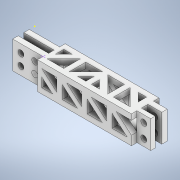
# Autodesk Inventor part: Final design
Saved by Autodesk Inventor 2021 (Build 250183000, 183)
## iProperties
Created: 2021-03-23
Part Number: Final design
Material: ABS Plastic
Document SubType Name: Modeling
Designer: kcf23
Mass: 34.1575 g
Surface Area: 224.112 cm^2
Volume: 32.224 cm^3
Density: 1.06 g/cm^3
Appearance: Smooth - White
Author: kcf23
Autodesk Inventor part; units mm, degrees
ref_plane "YZ Plane" through (0, 0, 0) normal (1, 0, 0) x (0, 1, 0)
ref_plane "XZ Plane" through (0, 0, 0) normal (0, 1, 0) x (-1, 0, 0)
ref_plane "XY Plane" through (0, 0, 0) normal (0, 0, 1) x (1, 0, 0)
sketch "Sketch1" plane through (0, 0, 0) normal (0, 0, 1) x (1, 0, 0)
  line L0 (0, 0) -> (127, 0)
  line L1 (127, 0) -> (127, 25.4)
  line L2 (127, 25.4) -> (0, 25.4)
  line L3 (0, 25.4) -> (0, 0)
  line L4 (0, 0) -> (12.7, 0)
  line L5 (12.7, 25.4) -> (0, 25.4)
  line L6 (0, 25.4) -> (0, 0)
  line L7 (7.62, 25.4) -> (0, 25.4)
  line L8 (0, 25.4) -> (0, -8.7611)
  line L9 (125.2545, 0) -> (125.2545, 25.4)
  circle A0 centre (121.4445, 4.9881) radius 2.2479
  circle A1 centre (121.4445, 12.6081) radius 2.2479
  circle A2 centre (121.4445, 20.2281) radius 2.2479
  line L10 (125.2545, 0) -> (117.6345, 0)
  line L11 (117.6345, 0) -> (117.6345, 25.4)
  line L12 (125.2545, 25.4) -> (117.6345, 25.4)
  line L13 (21.1145, 0) -> (21.1145, 25.4)
  circle A3 centre (5.08, 6.985) radius 2.2479
  line L14 (5.08, 6.985) -> (17.78, 6.985)
  circle A4 centre (17.78, 6.985) radius 2.2479
  circle A5 centre (5.08, 19.05) radius 2.2479
  line L15 (5.08, 19.05) -> (17.78, 19.05)
  circle A6 centre (17.78, 19.05) radius 2.2479
  line L16 (27.9985, 5.08) -> (27.9985, 20.32)
  line L17 (27.9985, 5.08) -> (45.7785, 5.08)
  line L18 (45.7785, 5.08) -> (45.7785, 20.32)
  line L19 (45.7785, 20.32) -> (27.9985, 20.32)
  line L20 (27.9985, 20.32) -> (27.9985, 5.08)
  line L21 (50.8, 20.32) -> (68.58, 20.32)
  line L22 (68.58, 20.32) -> (68.58, 5.08)
  line L23 (68.58, 5.08) -> (50.8, 5.08)
  line L24 (50.8, 5.08) -> (50.8, 20.32)
  line L25 (73.66, 5.08) -> (91.44, 5.08)
  line L26 (91.44, 5.08) -> (91.44, 20.32)
  line L27 (91.44, 20.32) -> (73.66, 20.32)
  line L28 (73.66, 20.32) -> (73.66, 5.08)
  line L29 (96.52, 20.32) -> (114.3, 20.32)
  line L30 (114.3, 20.32) -> (114.3, 5.08)
  line L31 (114.3, 5.08) -> (96.52, 5.08)
  line L32 (96.52, 5.08) -> (96.52, 20.32)
  line L33 (27.9985, 20.32) -> (45.7785, 5.08)
  line L34 (50.8, 20.32) -> (68.58, 5.08)
  line L35 (73.66, 20.32) -> (91.44, 5.08)
  line L36 (96.52, 20.32) -> (114.3, 5.08)
  line L37 (26.3455, 18.3915) -> (44.1255, 3.1515)
  line L38 (44.1255, 3.1515) -> (47.4315, 7.0085)
  line L39 (47.4315, 7.0085) -> (29.6515, 22.2485)
  line L40 (29.6515, 22.2485) -> (26.3455, 18.3915)
  line L41 (26.3455, 18.3915) -> (47.4315, 7.0085) construction
  line L42 (44.1255, 3.1515) -> (29.6515, 22.2485) construction
  line L43 (49.147, 18.3915) -> (66.927, 3.1515)
  line L44 (66.927, 3.1515) -> (70.233, 7.0085)
  line L45 (70.233, 7.0085) -> (52.453, 22.2485)
  line L46 (52.453, 22.2485) -> (49.147, 18.3915)
  line L47 (49.147, 18.3915) -> (70.233, 7.0085) construction
  line L48 (66.927, 3.1515) -> (52.453, 22.2485) construction
  line L49 (72.007, 18.3915) -> (89.787, 3.1515)
  line L50 (89.787, 3.1515) -> (93.093, 7.0085)
  line L51 (93.093, 7.0085) -> (75.313, 22.2485)
  line L52 (75.313, 22.2485) -> (72.007, 18.3915)
  line L53 (72.007, 18.3915) -> (93.093, 7.0085) construction
  line L54 (89.787, 3.1515) -> (75.313, 22.2485) construction
  line L55 (98.173, 22.2485) -> (115.953, 7.0085)
  line L56 (115.953, 7.0085) -> (112.647, 3.1515)
  line L57 (112.647, 3.1515) -> (94.867, 18.3915)
  line L58 (94.867, 18.3915) -> (98.173, 22.2485)
  line L59 (98.173, 22.2485) -> (112.647, 3.1515) construction
  line L60 (115.953, 7.0085) -> (94.867, 18.3915) construction
  line L61 (31.9015, 20.32) -> (31.9015, 5.08)
  point P0 (5.08, 5.6325)
  point P1 (5.08, 20.32)
  point P2 (6.5976, 20.3417)
  point P3 (36.8885, 12.7)
  point P4 (59.69, 12.7)
  point P5 (82.55, 12.7)
  point P6 (105.41, 12.7)
  point P7 (41.8756, 5.08)
  point P8 (27.9985, 16.9746)
  point P9 (114.3, 8.4254)
  point P10 (100.4229, 20.32)
  point P11 (91.44, 8.4254)
  point P12 (77.5629, 20.32)
  point P13 (68.58, 8.4254)
  point P14 (54.7029, 20.32)
  point P15 (110.3971, 5.08)
  point P16 (96.52, 16.9746)
  point P17 (87.5371, 5.08)
  point P18 (73.66, 16.9746)
  point P19 (64.6771, 5.08)
  point P20 (50.8, 16.9746)
  point P21 (45.7785, 8.4254)
  point P22 (31.9015, 13.6292)
  point P23 (5.08, 19.05)
  point P24 (17.78, 25.4)
  point P25 (17.78, 6.985)
  dimension "d0" = 127
  dimension "d1" = 25.4
  dimension "d20" = 25.4
  dimension "d21" = 4.4958
  dimension "d22" = 4.4958
  dimension "d23" = 4.4958
  dimension "d24" = 7.62
  dimension "d26" = 4.4958
  dimension "d27" = 12.7
  dimension "d28" = 4.4958
  dimension "d29" = 4.4958
  dimension "d30" = 12.7
  dimension "d31" = 4.4958
  dimension "d35" = 96.52
  dimension "d36" = 15.24
  dimension "d37" = 17.78
  dimension "d38" = 17.78
  dimension "d39" = 17.78
  dimension "d40" = 17.78
  dimension "d41" = 5.08
  dimension "d42" = 5.08
  dimension "d43" = 5.08
  dimension "d44" = 5.08
  constraints: 124 end point, 24 parallel, 14 point on line, 12 midpoint, 12 perpendicular, 8 horizontal, 7 centre point, 2 coincident, 1 collinear
  measures "d0" distance of L2.end L1.end
  measures "d1" distance of L1.end L0.end
  measures "d20" distance of L9.end L9.start
  measures "d21" diameter of A0
  measures "d22" diameter of A1
  measures "d23" diameter of A2
  measures "d24" distance of L9.start L10.end
  measures "d26" diameter of A3
  measures "d27" distance of L14.start L14.end
  measures "d28" diameter of A4
  measures "d29" diameter of A5
  measures "d30" distance of L15.start L15.end
  measures "d31" diameter of A6
  measures "d35" distance of L10.end L13.start
  measures "d36" distance of L16.start L16.end
  measures "d37" distance of L19.end L18.end
  measures "d38" distance of L22.end L23.end
  measures "d39" distance of L27.end L26.end
  measures "d40" distance of L30.end L31.end
  measures "d41" distance of L38.end L37.end
  measures "d42" distance of L44.end L43.end
  measures "d43" distance of L50.end L49.end
  measures "d44" distance of L55.end L56.end
extrude "Extrusion1" add sketch "Sketch1" along normal blind 25.4 contours L3 L2 L13 L0 | L13 L2 L11 L0 | L11 L2 L9 L0 | L9 L2 L1 L0 | L16 L37 L61 L17 | L37 L40 L16 | L16 L33 L61 L37 | L40 L39 L19 | L19 L61 L33 | L61 L33 L17 L37 | L17 L38 L37 | L39 L18 L33 L61 | L18 L39 L38 | L46 L45 L21 | L34 L23 L43 L24 | L21 L45 L22 L34 | L24 L43 L46 | L44 L43 L23 | L22 L45 L44 | L49 L28 L35 L25 | L25 L50 L49 | L49 L52 L28 | L35 L27 L51 L26 | L26 L51 L50 | L52 L51 L27 | L58 L55 L29 | L36 L31 L57 L32 | L29 L55 L30 L36 | L32 L57 L58 | L56 L57 L31 | L30 L55 L56
sketch "Sketch2" plane through (0, 25.4, 0) normal (0, 1, 0) x (1, 0, 0)
  line L0 (0, -25.4) -> (127, -25.4)
  line L1 (127, -25.4) -> (127, 0)
  line L2 (127, 0) -> (0, 0)
  line L3 (0, 0) -> (0, -25.4)
  line L4 (31.75, -20.32) -> (46.99, -20.32)
  line L5 (46.99, -20.32) -> (46.99, -5.08)
  line L6 (46.99, -5.08) -> (31.75, -20.32)
  line L7 (52.07, -20.32) -> (52.07, -5.08)
  line L8 (52.07, -5.08) -> (67.31, -5.08)
  line L9 (67.31, -5.08) -> (52.07, -20.32)
  line L10 (72.39, -5.08) -> (87.63, -5.08)
  line L11 (87.63, -5.08) -> (87.63, -20.32)
  line L12 (87.63, -20.32) -> (72.39, -5.08)
  line L13 (92.71, -5.08) -> (92.71, -20.32)
  line L14 (92.71, -20.32) -> (107.95, -20.32)
  line L15 (107.95, -20.32) -> (92.71, -5.08)
  line L16 (31.75, -5.08) -> (31.75, -12.7)
  line L17 (31.75, -5.08) -> (39.37, -5.08)
  line L18 (39.37, -5.08) -> (31.75, -12.7)
  line L19 (59.69, -20.32) -> (67.31, -20.32)
  line L20 (67.31, -20.32) -> (67.31, -12.7)
  line L21 (67.31, -12.7) -> (59.69, -20.32)
  line L22 (72.39, -20.32) -> (72.39, -12.7)
  line L23 (72.39, -20.32) -> (80.01, -20.32)
  line L24 (80.01, -20.32) -> (72.39, -12.7)
  line L25 (107.95, -12.7) -> (107.95, -5.08)
  line L26 (107.95, -5.08) -> (100.33, -5.08)
  line L27 (100.33, -5.08) -> (107.95, -12.7)
  line L28 (0, -25.4) -> (127, -25.4) projected
  point P0 (0, 0)
  point P1 (40.64, -20.32)
  dimension "d47" = 127
  dimension "d48" = 25.4
  dimension "d51" = 15.24
  dimension "d52" = 15.24
  dimension "d53" = 15.24
  dimension "d54" = 15.24
  dimension "d55" = 15.24
  dimension "d56" = 15.24
  dimension "d62" = 7.62
  dimension "d63" = 7.62
  dimension "d64" = 7.62
  constraints: 56 end point, 10 perpendicular, 4 point on line, 4 vertical, 3 horizontal, 2 parallel
  measures "d47" distance of L2.end L1.end
  measures "d48" distance of L0.end L1.end
  measures "d51" distance of L4.start L4.end
  measures "d52" distance of L4.end L5.end
  measures "d53" distance of L7.end L8.end
  measures "d54" distance of L10.start L10.end
  measures "d55" distance of L10.end L11.end
  measures "d56" distance of L13.end L14.end
  measures "d62" distance of L16.start L17.end
  measures "d63" distance of L19.end L20.end
  measures "d64" distance of L22.start L23.end
sketch "Sketch3" plane through (127, 0, 0) normal (1, 0, 0) x (0, 0, -1)
  line L0 (0, 20.32) -> (-25.4, 20.32) projected
  line L1 (-5.08, 5.08) -> (-20.32, 5.08)
  line L2 (-20.32, 5.08) -> (-20.32, 20.32)
  line L3 (-20.32, 20.32) -> (-5.08, 20.32)
  line L4 (-5.08, 20.32) -> (-5.08, 5.08)
  point P0 (0, 0)
  dimension "d65" = 15.24
  constraints: 8 end point, 2 parallel, 1 horizontal, 1 perpendicular, 1 point on line
  measures "d65" distance of L2.end L3.end
extrude "Extrusion2" cut sketch "Sketch3" against normal through all
sketch "Sketch5" plane through (0, 25.4, 0) normal (0, 1, 0) x (1, 0, 0)
  point P0 (0, 0)
sketch "Sketch6" plane through (0, 25.4, 0) normal (0, 1, 0) x (1, 0, 0)
  point P0 (0, 0)
  point P1 (27.94, -20.32)
extrude "Extrusion4" cut sketch "Sketch2" against normal through all contours L6 L5 L4 | L7 L8 L9 | L10 L11 L12 | L15 L14 L13 | L17 L18 L16 | L21 L20 L19 | L22 L24 L23 | L27 L26 L25
sketch "Sketch7" plane through (0, 0, 25.4) normal (0, 0, 1) x (1, 0, 0)
  line L0 (127, 0) -> (127, 25.4) projected
  line L1 (114.3, 20.32) -> (114.3, 8.4254) projected
  line L2 (0, 0) -> (127, 0) projected
  line L3 (120.65, 0) -> (120.65, 25.4)
  line L4 (127, 25.4) -> (0, 25.4) projected
  circle A0 centre (120.65, 19.05) radius 2.7432
  circle A1 centre (120.65, 6.35) radius 2.7432
  point P0 (121.4445, 12.6081)
  point P1 (121.4445, 20.2281)
  point P2 (121.4445, 4.9881)
  point P3 (120.65, 20.32)
  point P4 (120.65, 12.7)
  point P5 (120.65, 5.08)
  dimension "d84" = 12.7
  dimension "d108" = 5.4864
  dimension "d109" = 5.4864
  constraints: 6 point on line, 2 centre point, 2 end point, 1 midpoint, 1 vertical
  measures "d84" distance between parallel lines of L0 L1
  measures "d108" diameter of A0
  measures "d109" diameter of A1
sketch "Sketch8" plane through (0, 0, 0) normal (0, 0, -1) x (-1, 0, 0)
  line L0 (-127, 25.4) -> (0, 25.4) projected
  line L1 (-127, 0) -> (-127, 25.4) projected
  line L2 (-114.3, 25.4) -> (-127, 25.4)
  line L3 (-127, 25.4) -> (-127, 0)
  line L4 (-127, 0) -> (-114.3, 0)
  line L5 (-114.3, 0) -> (-114.3, 25.4)
  point P0 (0, 0)
  constraints: 8 end point, 2 parallel, 1 horizontal, 1 perpendicular, 1 point on line
extrude "Extrusion5" add sketch "Sketch8" against normal blind 25.4
sketch "Sketch9" plane through (0, 25.4, 0) normal (0, 1, 0) x (1, 0, 0)
  line L0 (127, 0) -> (127, -25.4) projected
  line L1 (114.3, -20.32) -> (110.3971, -20.32) projected
  line L2 (127, -5.08) -> (114.3, -5.08)
  line L3 (114.3, -5.08) -> (114.3, -20.32)
  line L4 (114.3, -20.32) -> (127, -20.32)
  line L5 (127, -20.32) -> (127, -5.08)
  line L6 (114.3, 0) -> (114.3, -5.08) projected
  line L7 (114.3, -5.08) -> (127, -5.08)
  line L8 (127, -5.08) -> (127, 0)
  line L9 (127, 0) -> (114.3, 0)
  line L10 (114.3, 0) -> (114.3, -5.08)
  line L11 (127, -20.32) -> (114.3, -20.32)
  line L12 (114.3, -20.32) -> (114.3, -25.4)
  line L13 (114.3, -25.4) -> (127, -25.4)
  line L14 (127, -25.4) -> (127, -20.32)
  line L15 (114.3, -5.08) -> (127, -5.08)
  line L16 (127, -5.08) -> (127, -10.16)
  line L17 (127, -10.16) -> (114.3, -10.16)
  line L18 (114.3, -10.16) -> (114.3, -5.08)
  line L19 (127, -20.32) -> (121.92, -20.32)
  line L20 (121.92, -20.32) -> (121.92, -16.2521)
  line L21 (121.92, -16.2521) -> (127, -16.2521)
  line L22 (127, -16.2521) -> (127, -20.32)
  line L23 (114.3, 0) -> (114.3, -25.4) projected
  line L24 (121.92, -20.32) -> (114.3, -20.32)
  line L25 (114.3, -20.32) -> (114.3, -16.2521)
  line L26 (114.3, -16.2521) -> (121.92, -16.2521)
  line L27 (121.92, -16.2521) -> (121.92, -20.32)
  point P0 (0, 0)
  dimension "d75" = 12.7
  dimension "d76" = 5.08
  dimension "d77" = 5.08
  constraints: 48 end point, 12 parallel, 6 horizontal, 6 perpendicular, 5 point on line
  measures "d75" distance of L4.end L1.start
  measures "d76" distance of L15.end L16.end
  measures "d77" distance of L20.end L21.end
sketch "Sketch11" plane through (0, 25.4, 25.4) normal (0, 1, 0) x (1, 0, 0)
  line L0 (0, 25.4) -> (0, 0) projected
  line L1 (0, 20.32) -> (27.94, 20.32)
  line L2 (27.94, 20.32) -> (27.94, 5.08)
  line L3 (27.94, 5.08) -> (0, 5.08)
  line L4 (0, 5.08) -> (0, 20.32)
  dimension "d90" = 27.94
  constraints: 8 end point, 2 parallel, 1 horizontal, 1 perpendicular, 1 point on line
  measures "d90" distance of L2.end L3.end
extrude "Extrusion10" add sketch "Sketch11" against normal blind 25.4
sketch "Sketch13" plane through (0, 25.4, 25.4) normal (0, 1, 0) x (1, 0, 0)
  line L0 (0, 25.4) -> (0, 0) projected
  line L1 (0, 10.16) -> (0, 15.24)
  line L2 (0, 10.16) -> (0, 15.24)
  line L3 (0, 15.24) -> (27.94, 15.24)
  line L4 (27.94, 15.24) -> (27.94, 10.16)
  line L5 (27.94, 10.16) -> (0, 10.16)
  line L6 (0, 25.4) -> (0, 0) projected
  dimension "d96" = 27.94
  constraints: 10 end point, 2 parallel, 2 point on line, 1 collinear, 1 perpendicular
  measures "d96" distance of L1.end L3.end
extrude "Extrusion12" cut sketch "Sketch13" against normal blind 25.4
sketch "Sketch14" plane through (0, 25.4, 25.4) normal (0, 1, 0) x (1, 0, 0)
  line L0 (0, 25.4) -> (127, 25.4) projected
  line L1 (27.94, 20.32) -> (27.94, 15.24) projected
  line L2 (0, 25.4) -> (27.94, 25.4)
  line L3 (27.94, 25.4) -> (27.94, 20.32)
  line L4 (27.94, 20.32) -> (0, 20.32)
  line L5 (0, 20.32) -> (0, 25.4)
  line L6 (127, 0) -> (0, 0) projected
  line L7 (0, 0) -> (27.94, 0)
  line L8 (27.94, 0) -> (27.94, 5.08)
  line L9 (27.94, 5.08) -> (0, 5.08)
  line L10 (0, 5.08) -> (0, 0)
  point P0 (114.3, 25.4)
  point P1 (114.3, 0)
  dimension "d99" = 5.08
  constraints: 16 end point, 4 parallel, 2 horizontal, 2 perpendicular
  measures "d99" distance of L8.end L7.end
extrude "Extrusion13" cut sketch "Sketch14" against normal through all
extrude "Extrusion15" cut sketch "Sketch9" against normal through all contours L0 L2 L6 L9 | L0 L21 L26 L3 L17 | L0 L13 L12 L4
extrude "Extrusion16" cut sketch "Sketch7" against normal through all contours A1 L3 | L3 A1 | A0 L3 | L3 A0
sketch "Sketch16" plane through (0, 0, 20.32) normal (0, 0, 1) x (1, 0, 0)
  line L0 (13.97, 17.78) -> (7.62, 17.78)
  line L1 (13.97, 17.78) -> (20.32, 17.78)
  circle A0 centre (7.62, 17.78) radius 2.7432
  circle A1 centre (20.32, 17.78) radius 2.7432
  line L2 (0, 0) -> (0, 25.4) projected
  line L3 (27.94, 25.4) -> (27.94, 0) projected
  line L4 (0, 25.4) -> (27.94, 25.4) projected
  line L5 (13.97, 7.62) -> (7.62, 7.62)
  line L6 (13.97, 7.62) -> (20.32, 7.62)
  circle A2 centre (7.62, 7.62) radius 2.7432
  circle A3 centre (20.32, 7.62) radius 2.7432
  dimension "d112" = 6.35
  dimension "d113" = 6.35
  dimension "d114" = 5.4864
  dimension "d115" = 5.4864
  dimension "d116" = 7.62
  dimension "d117" = 7.62
  dimension "d118" = 7.62
  dimension "d119" = 6.35
  dimension "d120" = 6.35
  dimension "d121" = 5.4864
  dimension "d122" = 5.4864
  constraints: 8 end point, 4 centre point, 4 coincident, 4 horizontal
  measures "d112" distance of L0.start L0.end
  measures "d113" distance of L0.start L1.end
  measures "d114" diameter of A0
  measures "d115" diameter of A1
  measures "d116" distance from line of L2 L0.end
  measures "d117" distance from line of L3 L1.end
  measures "d118" distance from line of L4 L0.end
  measures "d119" distance of L5.start L5.end
  measures "d120" distance of L5.start L6.end
  measures "d121" diameter of A2
  measures "d122" diameter of A3
extrude "Extrusion17" cut sketch "Sketch16" against normal through all
body "Solid1"
